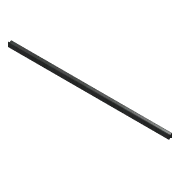
# Autodesk Inventor part: Track
Saved by Autodesk Inventor 2016 (Build 200138000, 138)
## iProperties
Created: 2015-05-19
Part Number: Track
Material: Steel
Document SubType Name: Modeling
Designer: Andy
Mass: 1513.73 g
Surface Area: 580.829 cm^2
Volume: 192.832 cm^3
Density: 7.85 g/cm^3
Appearance: Plate
Author: Andy
Autodesk Inventor part; units mm, degrees
ref_plane "YZ Plane" through (0, 0, 0) normal (1, 0, 0) x (0, 1, 0)
ref_plane "XZ Plane" through (0, 0, 0) normal (0, 1, 0) x (-1, 0, 0)
ref_plane "XY Plane" through (0, 0, 0) normal (0, 0, 1) x (1, 0, 0)
sketch "Sketch1" plane through (0, 0, 0) normal (1, 0, 0) x (0, 1, 0)
  line L0 (-15, 19.9) -> (-15, 0)
  line L1 (-15, 0) -> (-11.5, 0)
  line L2 (-11.5, 0) -> (-8.2, 4.25)
  line L3 (-11.5, 19.9) -> (-8.2, 15.65)
  line L4 (-11.5, 19.9) -> (-15, 19.9)
  line L5 (0, 19.9) -> (-1.5, 19.9)
  line L6 (-1.5, 19.9) -> (-8.2, 15.65)
  line L7 (-1.5, 0) -> (-8.2, 4.25)
  line L8 (0, 0) -> (-1.5, 0)
  line L9 (0, 19.9) -> (0, 0)
  point P0 (0, 0)
  dimension "d9" = 1.5
  dimension "d10" = 1.5
  constraints: 20 end point, 1 horizontal, 1 vertical
  measures "d9" distance of L5.start L5.end
  measures "d10" distance of L8.start L7.start
extrude "Extrusion1" add sketch "Sketch1" along normal blind 753.25
body "Solid1"
